Autodesk Inventor part; units mm, degrees
(part 2 of 5)
  spline S286 degree 2 poles (22.7063, 9.669) (22.5993, 9.5961) (22.4048, 9.5296) (22.2897, 9.5296) knots 0 0 0 1 2 2 2
  spline S287 degree 2 poles (22.2897, 9.5296) (22.1795, 9.5296) (21.9964, 9.5782) (21.904, 9.6479) knots 0 0 0 1 2 2 2
  spline S288 degree 2 poles (21.904, 9.6479) (21.797, 9.7306) (21.6868, 9.9818) (21.6868, 10.1585) knots 0 0 0 1 2 2 2
  spline S289 degree 2 poles (22.7128, 9.9883) (22.7128, 10.1909) (22.6382, 10.447) (22.5718, 10.5167) knots 0 0 0 1 2 2 2
  spline S290 degree 2 poles (22.5718, 10.5167) (22.5134, 10.5815) (22.3919, 10.6301) (22.3205, 10.6301) knots 0 0 0 1 2 2 2
  spline S291 degree 2 poles (22.3205, 10.6301) (22.1552, 10.6301) (21.9591, 10.3935) (21.9591, 10.1698) knots 0 0 0 1 2 2 2
  spline S292 degree 2 poles (21.9591, 10.1698) (21.9591, 10.0434) (22.0239, 9.8797) (22.0953, 9.8214) knots 0 0 0 1 2 2 2
  spline S293 degree 2 poles (22.0953, 9.8214) (22.1471, 9.7792) (22.2752, 9.7517) (22.3497, 9.7517) knots 0 0 0 1 2 2 2
  spline S294 degree 2 poles (22.3497, 9.7517) (22.4356, 9.7517) (22.6333, 9.8116) (22.7079, 9.8619) knots 0 0 0 1 2 2 2
  spline S295 degree 2 poles (22.7079, 9.8619) (22.7095, 9.8813) (22.7128, 9.9478) (22.7128, 9.9883) knots 0 0 0 1 2 2 2
  line L268 (24.0742, 10.8975) -> (23.2914, 8.374)
  line L269 (23.2914, 8.374) -> (23.0645, 8.374)
  line L270 (23.0645, 8.374) -> (23.844, 10.8975)
  line L271 (23.844, 10.8975) -> (24.0742, 10.8975)
  line L272 (25.528, 8.8084) -> (24.2946, 8.8084)
  line L273 (24.2946, 8.8084) -> (24.2946, 9.092)
  spline S296 degree 2 poles (24.2946, 9.092) (24.4275, 9.2168) (24.6641, 9.4486) (24.7776, 9.5734) knots 0 0 0 1 2 2 2
  spline S297 degree 2 poles (24.7776, 9.5734) (25.0061, 9.8246) (25.1731, 10.1261) (25.1731, 10.2865) knots 0 0 0 1 2 2 2
  spline S298 degree 2 poles (25.1731, 10.2865) (25.1731, 10.3708) (25.1212, 10.4972) (25.0742, 10.5377) knots 0 0 0 1 2 2 2
  spline S299 degree 2 poles (25.0742, 10.5377) (25.0272, 10.5782) (24.904, 10.6188) (24.8295, 10.6188) knots 0 0 0 1 2 2 2
  spline S300 degree 2 poles (24.8295, 10.6188) (24.7581, 10.6188) (24.6123, 10.5831) (24.5458, 10.5555) knots 0 0 0 1 2 2 2
  spline S301 degree 2 poles (24.5458, 10.5555) (24.4891, 10.5329) (24.3837, 10.468) (24.3513, 10.4453) knots 0 0 0 1 2 2 2
  line L274 (24.3513, 10.4453) -> (24.3367, 10.4453)
  line L275 (24.3367, 10.4453) -> (24.3367, 10.7306)
  spline S302 degree 2 poles (24.3367, 10.7306) (24.4194, 10.7711) (24.716, 10.8505) (24.8489, 10.8505) knots 0 0 0 1 2 2 2
  spline S303 degree 2 poles (24.8489, 10.8505) (25.1293, 10.8505) (25.4453, 10.5539) (25.4453, 10.3011) knots 0 0 0 1 2 2 2
  spline S304 degree 2 poles (25.4453, 10.3011) (25.4453, 10.1828) (25.3902, 9.985) (25.3416, 9.9008) knots 0 0 0 1 2 2 2
  spline S305 degree 2 poles (25.3416, 9.9008) (25.293, 9.8132) (25.152, 9.6414) (25.0742, 9.5588) knots 0 0 0 1 2 2 2
  spline S306 degree 2 poles (25.0742, 9.5588) (24.9478, 9.421) (24.6382, 9.1261) (24.5458, 9.0402) knots 0 0 0 1 2 2 2
  line L276 (24.5458, 9.0402) -> (25.528, 9.0402)
  line L277 (25.528, 9.0402) -> (25.528, 8.8084)
  spline S307 degree 2 poles (27.0401, 9.8084) (27.0401, 9.2703) (26.7273, 8.7662) (26.4016, 8.7662) knots 0 0 0 1 2 2 2
  spline S308 degree 2 poles (26.4016, 8.7662) (26.0709, 8.7662) (25.7614, 9.28) (25.7614, 9.8068) knots 0 0 0 1 2 2 2
  spline S309 degree 2 poles (25.7614, 9.8068) (25.7614, 10.3481) (26.0742, 10.8489) (26.4016, 10.8489) knots 0 0 0 1 2 2 2
  spline S310 degree 2 poles (26.4016, 10.8489) (26.7306, 10.8489) (27.0401, 10.3303) (27.0401, 9.8084) knots 0 0 0 1 2 2 2
  spline S311 degree 2 poles (26.6966, 9.199) (26.7354, 9.2978) (26.7679, 9.6026) (26.7679, 9.8084) knots 0 0 0 1 2 2 2
  spline S312 degree 2 poles (26.7679, 9.8084) (26.7679, 10.0142) (26.7354, 10.3173) (26.6949, 10.4194) knots 0 0 0 1 2 2 2
  spline S313 degree 2 poles (26.6949, 10.4194) (26.6544, 10.5215) (26.5134, 10.6269) (26.4016, 10.6269) knots 0 0 0 1 2 2 2
  spline S314 degree 2 poles (26.4016, 10.6269) (26.2897, 10.6269) (26.1455, 10.5215) (26.1034, 10.4162) knots 0 0 0 1 2 2 2
  spline S315 degree 2 poles (26.1034, 10.4162) (26.0628, 10.3141) (26.0337, 10.0029) (26.0337, 9.8068) knots 0 0 0 1 2 2 2
  spline S316 degree 2 poles (26.0337, 9.8068) (26.0337, 9.5961) (26.0596, 9.3141) (26.1017, 9.2038) knots 0 0 0 1 2 2 2
  spline S317 degree 2 poles (26.1017, 9.2038) (26.1406, 9.1001) (26.2849, 8.9883) (26.4016, 8.9883) knots 0 0 0 1 2 2 2
  spline S318 degree 2 poles (26.4016, 8.9883) (26.5118, 8.9883) (26.656, 9.0936) (26.6966, 9.199) knots 0 0 0 1 2 2 2
  spline S319 degree 2 poles (-27.8415, 6.1297) (-27.8415, 5.9806) (-27.955, 5.7521) (-28.049, 5.6775) knots 0 0 0 1 2 2 2
  spline S320 degree 2 poles (-28.049, 5.6775) (-28.1624, 5.59) (-28.4201, 5.5154) (-28.6244, 5.5154) knots 0 0 0 1 2 2 2
  line L278 (-28.6244, 5.5154) -> (-29.1981, 5.5154)
  line L279 (-29.1981, 5.5154) -> (-29.1981, 7.5154)
  line L280 (-29.1981, 7.5154) -> (-28.6681, 7.5154)
  spline S321 degree 2 poles (-28.6681, 7.5154) (-28.4542, 7.5154) (-28.2402, 7.4879) (-28.143, 7.4344) knots 0 0 0 1 2 2 2
  spline S322 degree 2 poles (-28.143, 7.4344) (-28.0344, 7.3777) (-27.9355, 7.1913) (-27.9355, 7.0649) knots 0 0 0 1 2 2 2
  spline S323 degree 2 poles (-27.9355, 7.0649) (-27.9355, 6.9239) (-28.0846, 6.7002) (-28.2159, 6.637) knots 0 0 0 1 2 2 2
  line L281 (-28.2159, 6.637) -> (-28.2159, 6.6273)
  spline S324 degree 2 poles (-28.2159, 6.6273) (-28.0376, 6.5786) (-27.8415, 6.3209) (-27.8415, 6.1297) knots 0 0 0 1 2 2 2
  spline S325 degree 2 poles (-28.1187, 6.1184) (-28.1187, 6.2318) (-28.1835, 6.3777) (-28.2808, 6.4295) knots 0 0 0 1 2 2 2
  spline S326 degree 2 poles (-28.2808, 6.4295) (-28.344, 6.462) (-28.4931, 6.4814) (-28.6308, 6.4814) knots 0 0 0 1 2 2 2
  line L282 (-28.6308, 6.4814) -> (-28.9323, 6.4814)
  line L283 (-28.9323, 6.4814) -> (-28.9323, 5.7423)
  line L284 (-28.9323, 5.7423) -> (-28.7167, 5.7423)
  spline S327 degree 2 poles (-28.7167, 5.7423) (-28.5417, 5.7423) (-28.3407, 5.7748) (-28.2629, 5.8266) knots 0 0 0 1 2 2 2
  spline S328 degree 2 poles (-28.2629, 5.8266) (-28.1884, 5.8801) (-28.1187, 6.013) (-28.1187, 6.1184) knots 0 0 0 1 2 2 2
  spline S329 degree 2 poles (-28.2127, 7.0276) (-28.2127, 7.0989) (-28.2613, 7.2059) (-28.3148, 7.2367) knots 0 0 0 1 2 2 2
  spline S330 degree 2 poles (-28.3148, 7.2367) (-28.3796, 7.2723) (-28.5368, 7.2885) (-28.6778, 7.2885) knots 0 0 0 1 2 2 2
  line L285 (-28.6778, 7.2885) -> (-28.9323, 7.2885)
  line L286 (-28.9323, 7.2885) -> (-28.9323, 6.7034)
  line L287 (-28.9323, 6.7034) -> (-28.6308, 6.7034)
  spline S331 degree 2 poles (-28.6308, 6.7034) (-28.506, 6.7034) (-28.3877, 6.7294) (-28.3245, 6.7699) knots 0 0 0 1 2 2 2
  spline S332 degree 2 poles (-28.3245, 6.7699) (-28.2629, 6.8088) (-28.2127, 6.9336) (-28.2127, 7.0276) knots 0 0 0 1 2 2 2
  spline S333 degree 2 poles (-26.7605, 5.6743) (-26.7913, 5.6516) (-26.895, 5.5705) (-26.9436, 5.5462) knots 0 0 0 1 2 2 2
  spline S334 degree 2 poles (-26.9436, 5.5462) (-27.0101, 5.5106) (-27.1349, 5.4733) (-27.2483, 5.4733) knots 0 0 0 1 2 2 2
  spline S335 degree 2 poles (-27.2483, 5.4733) (-27.3407, 5.4733) (-27.5077, 5.543) (-27.5709, 5.6062) knots 0 0 0 1 2 2 2
  spline S336 degree 2 poles (-27.5709, 5.6062) (-27.6308, 5.6678) (-27.7038, 5.8493) (-27.7038, 5.9498) knots 0 0 0 1 2 2 2
  spline S337 degree 2 poles (-27.7038, 5.9498) (-27.7038, 6.1054) (-27.5725, 6.3258) (-27.4299, 6.389) knots 0 0 0 1 2 2 2
  spline S338 degree 2 poles (-27.4299, 6.389) (-27.3034, 6.4474) (-26.9599, 6.4911) (-26.7605, 6.5025) knots 0 0 0 1 2 2 2
  line L288 (-26.7605, 6.5025) -> (-26.7605, 6.5511)
  spline S339 degree 2 poles (-26.7605, 6.5511) (-26.7605, 6.6386) (-26.814, 6.7472) (-26.8626, 6.778) knots 0 0 0 1 2 2 2
  spline S340 degree 2 poles (-26.8626, 6.778) (-26.9112, 6.8088) (-27.0506, 6.8282) (-27.1252, 6.8282) knots 0 0 0 1 2 2 2
  spline S341 degree 2 poles (-27.1252, 6.8282) (-27.2127, 6.8282) (-27.4493, 6.7764) (-27.5676, 6.7261) knots 0 0 0 1 2 2 2
  line L289 (-27.5676, 6.7261) -> (-27.5822, 6.7261)
  line L290 (-27.5822, 6.7261) -> (-27.5822, 6.9838)
  spline S342 degree 2 poles (-27.5822, 6.9838) (-27.5125, 7.0033) (-27.2516, 7.0519) (-27.1235, 7.0519) knots 0 0 0 1 2 2 2
  spline S343 degree 2 poles (-27.1235, 7.0519) (-26.968, 7.0519) (-26.7556, 7.0033) (-26.6714, 6.9401) knots 0 0 0 1 2 2 2
  spline S344 degree 2 poles (-26.6714, 6.9401) (-26.5887, 6.8785) (-26.5077, 6.6824) (-26.5077, 6.5414) knots 0 0 0 1 2 2 2
  line L291 (-26.5077, 6.5414) -> (-26.5077, 5.5154)
  line L292 (-26.5077, 5.5154) -> (-26.7605, 5.5154)
  line L293 (-26.7605, 5.5154) -> (-26.7605, 5.6743)
  line L294 (-26.7605, 5.885) -> (-26.7605, 6.3015)
  spline S345 degree 2 poles (-26.7605, 6.3015) (-26.8513, 6.2934) (-27.1252, 6.2658) (-27.2111, 6.2399) knots 0 0 0 1 2 2 2
  spline S346 degree 2 poles (-27.2111, 6.2399) (-27.3116, 6.2091) (-27.4428, 6.0811) (-27.4428, 5.9676) knots 0 0 0 1 2 2 2
  spline S347 degree 2 poles (-27.4428, 5.9676) (-27.4428, 5.838) (-27.297, 5.7067) (-27.1576, 5.7067) knots 0 0 0 1 2 2 2
  spline S348 degree 2 poles (-27.1576, 5.7067) (-27.0393, 5.7067) (-26.8448, 5.8088) (-26.7605, 5.885) knots 0 0 0 1 2 2 2
  line L295 (-24.9744, 5.5154) -> (-25.2273, 5.5154)
  line L296 (-25.2273, 5.5154) -> (-25.2273, 6.3712)
  spline S349 degree 2 poles (-25.2273, 6.3712) (-25.2273, 6.4749) (-25.2467, 6.6532) (-25.2759, 6.7067) knots 0 0 0 1 2 2 2
  spline S350 degree 2 poles (-25.2759, 6.7067) (-25.3067, 6.7634) (-25.4169, 6.8185) (-25.5109, 6.8185) knots 0 0 0 1 2 2 2
  spline S351 degree 2 poles (-25.5109, 6.8185) (-25.6049, 6.8185) (-25.8043, 6.718) (-25.8999, 6.637) knots 0 0 0 1 2 2 2
  line L297 (-25.8999, 6.637) -> (-25.8999, 5.5154)
  line L298 (-25.8999, 5.5154) -> (-26.1527, 5.5154)
  line L299 (-26.1527, 5.5154) -> (-26.1527, 7.0162)
  line L300 (-26.1527, 7.0162) -> (-25.8999, 7.0162)
  line L301 (-25.8999, 7.0162) -> (-25.8999, 6.8493)
  spline S352 degree 2 poles (-25.8999, 6.8493) (-25.7864, 6.9514) (-25.5676, 7.0584) (-25.4445, 7.0584) knots 0 0 0 1 2 2 2
  spline S353 degree 2 poles (-25.4445, 7.0584) (-25.224, 7.0584) (-24.9744, 6.7667) (-24.9744, 6.4895) knots 0 0 0 1 2 2 2
  line L302 (-24.9744, 6.4895) -> (-24.9744, 5.5154)
  spline S354 degree 2 poles (-24.0231, 5.4814) (-24.1787, 5.4814) (-24.4364, 5.577) (-24.5287, 5.6743) knots 0 0 0 1 2 2 2
  spline S355 degree 2 poles (-24.5287, 5.6743) (-24.6211, 5.7699) (-24.7232, 6.0649) (-24.7232, 6.2626) knots 0 0 0 1 2 2 2
  spline S356 degree 2 poles (-24.7232, 6.2626) (-24.7232, 6.4603) (-24.6179, 6.7488) (-24.5287, 6.8461) knots 0 0 0 1 2 2 2
  spline S357 degree 2 poles (-24.5287, 6.8461) (-24.4396, 6.9449) (-24.1754, 7.0503) (-24.0231, 7.0503) knots 0 0 0 1 2 2 2
  spline S358 degree 2 poles (-24.0231, 7.0503) (-23.8999, 7.0503) (-23.6697, 6.9806) (-23.5806, 6.9352) knots 0 0 0 1 2 2 2
  line L303 (-23.5806, 6.9352) -> (-23.5806, 6.6516)
  line L304 (-23.5806, 6.6516) -> (-23.5952, 6.6516)
  spline S359 degree 2 poles (-23.5952, 6.6516) (-23.6227, 6.6743) (-23.707, 6.7326) (-23.767, 6.7634) knots 0 0 0 1 2 2 2
  spline S360 degree 2 poles (-23.767, 6.7634) (-23.8205, 6.7893) (-23.9631, 6.8299) (-24.0279, 6.8299) knots 0 0 0 1 2 2 2
  spline S361 degree 2 poles (-24.0279, 6.8299) (-24.224, 6.8299) (-24.4623, 6.5333) (-24.4623, 6.2626) knots 0 0 0 1 2 2 2
  spline S362 degree 2 poles (-24.4623, 6.2626) (-24.4623, 5.9984) (-24.2321, 5.7018) (-24.0279, 5.7018) knots 0 0 0 1 2 2 2
  spline S363 degree 2 poles (-24.0279, 5.7018) (-23.9047, 5.7018) (-23.6811, 5.8039) (-23.5952, 5.8833) knots 0 0 0 1 2 2 2
  line L305 (-23.5952, 5.8833) -> (-23.5806, 5.8833)
  line L306 (-23.5806, 5.8833) -> (-23.5806, 5.5997)
  spline S364 degree 2 poles (-23.5806, 5.5997) (-23.6179, 5.5819) (-23.7313, 5.5316) (-23.7767, 5.5203) knots 0 0 0 1 2 2 2
  spline S365 degree 2 poles (-23.7767, 5.5203) (-23.8415, 5.5009) (-23.9436, 5.4814) (-24.0231, 5.4814) knots 0 0 0 1 2 2 2
  spline S366 degree 2 poles (-22.1171, 6.2658) (-22.1171, 5.8866) (-22.4817, 5.4733) (-22.7864, 5.4733) knots 0 0 0 1 2 2 2
  spline S367 degree 2 poles (-22.7864, 5.4733) (-23.0992, 5.4733) (-23.4574, 5.8996) (-23.4574, 6.2658) knots 0 0 0 1 2 2 2
  spline S368 degree 2 poles (-23.4574, 6.2658) (-23.4574, 6.6419) (-23.0879, 7.0584) (-22.7864, 7.0584) knots 0 0 0 1 2 2 2
  spline S369 degree 2 poles (-22.7864, 7.0584) (-22.4817, 7.0584) (-22.1171, 6.6435) (-22.1171, 6.2658) knots 0 0 0 1 2 2 2
  spline S370 degree 2 poles (-22.378, 6.2658) (-22.378, 6.5576) (-22.5903, 6.8412) (-22.7864, 6.8412) knots 0 0 0 1 2 2 2
  spline S371 degree 2 poles (-22.7864, 6.8412) (-22.9825, 6.8412) (-23.1965, 6.5576) (-23.1965, 6.2658) knots 0 0 0 1 2 2 2
  spline S372 degree 2 poles (-23.1965, 6.2658) (-23.1965, 5.9822) (-22.9825, 5.6905) (-22.7864, 5.6905) knots 0 0 0 1 2 2 2
  spline S373 degree 2 poles (-22.7864, 5.6905) (-22.5919, 5.6905) (-22.378, 5.9774) (-22.378, 6.2658) knots 0 0 0 1 2 2 2
  line L307 (-19.8448, 5.5154) -> (-20.0976, 5.5154)
  line L308 (-20.0976, 5.5154) -> (-20.0976, 5.6678)
  spline S374 degree 2 poles (-20.0976, 5.6678) (-20.156, 5.6192) (-20.2419, 5.5543) (-20.3002, 5.5268) knots 0 0 0 1 2 2 2
  spline S375 degree 2 poles (-20.3002, 5.5268) (-20.3537, 5.5009) (-20.4688, 5.4733) (-20.5449, 5.4733) knots 0 0 0 1 2 2 2
  spline S376 degree 2 poles (-20.5449, 5.4733) (-20.6681, 5.4733) (-20.8756, 5.5754) (-20.9485, 5.6743) knots 0 0 0 1 2 2 2
  spline S377 degree 2 poles (-20.9485, 5.6743) (-21.0214, 5.7731) (-21.1025, 6.0649) (-21.1025, 6.2545) knots 0 0 0 1 2 2 2
  spline S378 degree 2 poles (-21.1025, 6.2545) (-21.1025, 6.4522) (-21.0004, 6.7407) (-20.9112, 6.8493) knots 0 0 0 1 2 2 2
  spline S379 degree 2 poles (-20.9112, 6.8493) (-20.8286, 6.9466) (-20.5968, 7.0584) (-20.4688, 7.0584) knots 0 0 0 1 2 2 2
  spline S380 degree 2 poles (-20.4688, 7.0584) (-20.3569, 7.0584) (-20.19, 7.0081) (-20.0976, 6.9563) knots 0 0 0 1 2 2 2
  line L309 (-20.0976, 6.9563) -> (-20.0976, 7.6046)
  line L310 (-20.0976, 7.6046) -> (-19.8448, 7.6046)
  line L311 (-19.8448, 7.6046) -> (-19.8448, 5.5154)
  line L312 (-20.0976, 5.8801) -> (-20.0976, 6.7472)
  spline S381 degree 2 poles (-20.0976, 6.7472) (-20.1916, 6.7926) (-20.3407, 6.8266) (-20.4266, 6.8266) knots 0 0 0 1 2 2 2
  spline S382 degree 2 poles (-20.4266, 6.8266) (-20.6211, 6.8266) (-20.8415, 6.5349) (-20.8415, 6.2594) knots 0 0 0 1 2 2 2
  spline S383 degree 2 poles (-20.8415, 6.2594) (-20.8415, 5.9936) (-20.673, 5.7132) (-20.4866, 5.7132) knots 0 0 0 1 2 2 2
  spline S384 degree 2 poles (-20.4866, 5.7132) (-20.3877, 5.7132) (-20.1868, 5.8039) (-20.0976, 5.8801) knots 0 0 0 1 2 2 2
  line L313 (-19.2208, 5.5154) -> (-19.4736, 5.5154)
  line L314 (-19.4736, 5.5154) -> (-19.4736, 7.0162)
  line L315 (-19.4736, 7.0162) -> (-19.2208, 7.0162)
  line L316 (-19.2208, 7.0162) -> (-19.2208, 5.5154)
  line L317 (-19.203, 7.2658) -> (-19.4898, 7.2658)
  line L318 (-19.4898, 7.2658) -> (-19.4898, 7.5284)
  line L319 (-19.4898, 7.5284) -> (-19.203, 7.5284)
  line L320 (-19.203, 7.5284) -> (-19.203, 7.2658)
  spline S385 degree 2 poles (-16.7329, 6.3064) (-16.7329, 5.9303) (-17.0911, 5.4863) (-17.365, 5.4863) knots 0 0 0 1 2 2 2
  spline S386 degree 2 poles (-17.365, 5.4863) (-17.4769, 5.4863) (-17.6487, 5.5381) (-17.7378, 5.5916) knots 0 0 0 1 2 2 2
  line L321 (-17.7378, 5.5916) -> (-17.7378, 4.9628)
  line L322 (-17.7378, 4.9628) -> (-17.9906, 4.9628)
  line L323 (-17.9906, 4.9628) -> (-17.9906, 7.0162)
  line L324 (-17.9906, 7.0162) -> (-17.7378, 7.0162)
  line L325 (-17.7378, 7.0162) -> (-17.7378, 6.859)
  spline S387 degree 2 poles (-17.7378, 6.859) (-17.6438, 6.9449) (-17.4137, 7.0584) (-17.2791, 7.0584) knots 0 0 0 1 2 2 2
  spline S388 degree 2 poles (-17.2791, 7.0584) (-17.0214, 7.0584) (-16.7329, 6.65) (-16.7329, 6.3064) knots 0 0 0 1 2 2 2
  spline S389 degree 2 poles (-16.9939, 6.2772) (-16.9939, 6.5349) (-17.1576, 6.8185) (-17.3407, 6.8185) knots 0 0 0 1 2 2 2
  spline S390 degree 2 poles (-17.3407, 6.8185) (-17.4477, 6.8185) (-17.6487, 6.7229) (-17.7378, 6.6483) knots 0 0 0 1 2 2 2
  line L326 (-17.7378, 6.6483) -> (-17.7378, 5.7958)
  spline S391 degree 2 poles (-17.7378, 5.7958) (-17.6389, 5.7488) (-17.4979, 5.7132) (-17.4072, 5.7132) knots 0 0 0 1 2 2 2
  spline S392 degree 2 poles (-17.4072, 5.7132) (-17.2111, 5.7132) (-16.9939, 6.0017) (-16.9939, 6.2772) knots 0 0 0 1 2 2 2
  line L327 (-15.6746, 6.7456) -> (-15.6876, 6.7456)
  spline S393 degree 2 poles (-15.6876, 6.7456) (-15.7167, 6.7537) (-15.7799, 6.7569) (-15.8237, 6.7569) knots 0 0 0 1 2 2 2
  spline S394 degree 2 poles (-15.8237, 6.7569) (-15.9258, 6.7569) (-16.1268, 6.6678) (-16.2175, 6.5803) knots 0 0 0 1 2 2 2
  line L328 (-16.2175, 6.5803) -> (-16.2175, 5.5154)
  line L329 (-16.2175, 5.5154) -> (-16.4704, 5.5154)
  line L330 (-16.4704, 5.5154) -> (-16.4704, 7.0162)
  line L331 (-16.4704, 7.0162) -> (-16.2175, 7.0162)
  line L332 (-16.2175, 7.0162) -> (-16.2175, 6.7926)
  spline S395 degree 2 poles (-16.2175, 6.7926) (-16.0798, 6.9158) (-15.874, 7.0162) (-15.7767, 7.0162) knots 0 0 0 1 2 2 2
  spline S396 degree 2 poles (-15.7767, 7.0162) (-15.7378, 7.0162) (-15.6989, 7.013) (-15.6746, 7.0081) knots 0 0 0 1 2 2 2
  line L333 (-15.6746, 7.0081) -> (-15.6746, 6.7456)
  spline S397 degree 2 poles (-14.2451, 6.2658) (-14.2451, 5.8866) (-14.6098, 5.4733) (-14.9145, 5.4733) knots 0 0 0 1 2 2 2
  spline S398 degree 2 poles (-14.9145, 5.4733) (-15.2273, 5.4733) (-15.5855, 5.8996) (-15.5855, 6.2658) knots 0 0 0 1 2 2 2
  spline S399 degree 2 poles (-15.5855, 6.2658) (-15.5855, 6.6419) (-15.2159, 7.0584) (-14.9145, 7.0584) knots 0 0 0 1 2 2 2
  spline S400 degree 2 poles (-14.9145, 7.0584) (-14.6098, 7.0584) (-14.2451, 6.6435) (-14.2451, 6.2658) knots 0 0 0 1 2 2 2
  spline S401 degree 2 poles (-14.506, 6.2658) (-14.506, 6.5576) (-14.7184, 6.8412) (-14.9145, 6.8412) knots 0 0 0 1 2 2 2
  spline S402 degree 2 poles (-14.9145, 6.8412) (-15.1106, 6.8412) (-15.3245, 6.5576) (-15.3245, 6.2658) knots 0 0 0 1 2 2 2
  spline S403 degree 2 poles (-15.3245, 6.2658) (-15.3245, 5.9822) (-15.1106, 5.6905) (-14.9145, 5.6905) knots 0 0 0 1 2 2 2
  spline S404 degree 2 poles (-14.9145, 5.6905) (-14.72, 5.6905) (-14.506, 5.9774) (-14.506, 6.2658) knots 0 0 0 1 2 2 2
  line L334 (-12.8075, 7.0162) -> (-13.3731, 5.5154)
  line L335 (-13.3731, 5.5154) -> (-13.6, 5.5154)
  line L336 (-13.6, 5.5154) -> (-14.1608, 7.0162)
  line L337 (-14.1608, 7.0162) -> (-13.8869, 7.0162)
  line L338 (-13.8869, 7.0162) -> (-13.4769, 5.8607)
  line L339 (-13.4769, 5.8607) -> (-13.0701, 7.0162)
  line L340 (-13.0701, 7.0162) -> (-12.8075, 7.0162)
  spline S405 degree 2 poles (-11.7799, 5.6743) (-11.8107, 5.6516) (-11.9145, 5.5705) (-11.9631, 5.5462) knots 0 0 0 1 2 2 2
  spline S406 degree 2 poles (-11.9631, 5.5462) (-12.0295, 5.5106) (-12.1543, 5.4733) (-12.2678, 5.4733) knots 0 0 0 1 2 2 2
  spline S407 degree 2 poles (-12.2678, 5.4733) (-12.3602, 5.4733) (-12.5271, 5.543) (-12.5903, 5.6062) knots 0 0 0 1 2 2 2
  spline S408 degree 2 poles (-12.5903, 5.6062) (-12.6503, 5.6678) (-12.7232, 5.8493) (-12.7232, 5.9498) knots 0 0 0 1 2 2 2
  spline S409 degree 2 poles (-12.7232, 5.9498) (-12.7232, 6.1054) (-12.5919, 6.3258) (-12.4493, 6.389) knots 0 0 0 1 2 2 2
  spline S410 degree 2 poles (-12.4493, 6.389) (-12.3229, 6.4474) (-11.9793, 6.4911) (-11.7799, 6.5025) knots 0 0 0 1 2 2 2
  line L341 (-11.7799, 6.5025) -> (-11.7799, 6.5511)
  spline S411 degree 2 poles (-11.7799, 6.5511) (-11.7799, 6.6386) (-11.8334, 6.7472) (-11.8821, 6.778) knots 0 0 0 1 2 2 2
  spline S412 degree 2 poles (-11.8821, 6.778) (-11.9307, 6.8088) (-12.0701, 6.8282) (-12.1446, 6.8282) knots 0 0 0 1 2 2 2
  spline S413 degree 2 poles (-12.1446, 6.8282) (-12.2321, 6.8282) (-12.4688, 6.7764) (-12.5871, 6.7261) knots 0 0 0 1 2 2 2
  line L342 (-12.5871, 6.7261) -> (-12.6017, 6.7261)
  line L343 (-12.6017, 6.7261) -> (-12.6017, 6.9838)
  spline S414 degree 2 poles (-12.6017, 6.9838) (-12.532, 7.0033) (-12.271, 7.0519) (-12.143, 7.0519) knots 0 0 0 1 2 2 2
  spline S415 degree 2 poles (-12.143, 7.0519) (-11.9874, 7.0519) (-11.7751, 7.0033) (-11.6908, 6.9401) knots 0 0 0 1 2 2 2
  spline S416 degree 2 poles (-11.6908, 6.9401) (-11.6081, 6.8785) (-11.5271, 6.6824) (-11.5271, 6.5414) knots 0 0 0 1 2 2 2
  line L344 (-11.5271, 6.5414) -> (-11.5271, 5.5154)
  line L345 (-11.5271, 5.5154) -> (-11.7799, 5.5154)
  line L346 (-11.7799, 5.5154) -> (-11.7799, 5.6743)
  line L347 (-11.7799, 5.885) -> (-11.7799, 6.3015)
  spline S417 degree 2 poles (-11.7799, 6.3015) (-11.8707, 6.2934) (-12.1446, 6.2658) (-12.2305, 6.2399) knots 0 0 0 1 2 2 2
  spline S418 degree 2 poles (-12.2305, 6.2399) (-12.331, 6.2091) (-12.4623, 6.0811) (-12.4623, 5.9676) knots 0 0 0 1 2 2 2
  spline S419 degree 2 poles (-12.4623, 5.9676) (-12.4623, 5.838) (-12.3164, 5.7067) (-12.177, 5.7067) knots 0 0 0 1 2 2 2
  spline S420 degree 2 poles (-12.177, 5.7067) (-12.0587, 5.7067) (-11.8642, 5.8088) (-11.7799, 5.885) knots 0 0 0 1 2 2 2
  spline S421 degree 2 poles (-9.0555, 6.3064) (-9.0555, 5.9303) (-9.4137, 5.4863) (-9.6876, 5.4863) knots 0 0 0 1 2 2 2
  spline S422 degree 2 poles (-9.6876, 5.4863) (-9.7994, 5.4863) (-9.9712, 5.5381) (-10.0603, 5.5916) knots 0 0 0 1 2 2 2
  line L348 (-10.0603, 5.5916) -> (-10.0603, 4.9628)
  line L349 (-10.0603, 4.9628) -> (-10.3132, 4.9628)
  line L350 (-10.3132, 4.9628) -> (-10.3132, 7.0162)
  line L351 (-10.3132, 7.0162) -> (-10.0603, 7.0162)
  line L352 (-10.0603, 7.0162) -> (-10.0603, 6.859)
  spline S423 degree 2 poles (-10.0603, 6.859) (-9.9663, 6.9449) (-9.7362, 7.0584) (-9.6017, 7.0584) knots 0 0 0 1 2 2 2
  spline S424 degree 2 poles (-9.6017, 7.0584) (-9.344, 7.0584) (-9.0555, 6.65) (-9.0555, 6.3064) knots 0 0 0 1 2 2 2
  spline S425 degree 2 poles (-9.3164, 6.2772) (-9.3164, 6.5349) (-9.4801, 6.8185) (-9.6633, 6.8185) knots 0 0 0 1 2 2 2
  spline S426 degree 2 poles (-9.6633, 6.8185) (-9.7702, 6.8185) (-9.9712, 6.7229) (-10.0603, 6.6483) knots 0 0 0 1 2 2 2
  line L353 (-10.0603, 6.6483) -> (-10.0603, 5.7958)
  spline S427 degree 2 poles (-10.0603, 5.7958) (-9.9615, 5.7488) (-9.8205, 5.7132) (-9.7297, 5.7132) knots 0 0 0 1 2 2 2
  spline S428 degree 2 poles (-9.7297, 5.7132) (-9.5336, 5.7132) (-9.3164, 6.0017) (-9.3164, 6.2772) knots 0 0 0 1 2 2 2
  spline S429 degree 2 poles (-8.1414, 5.4814) (-8.5012, 5.4814) (-8.8966, 5.885) (-8.8966, 6.2577) knots 0 0 0 1 2 2 2
  spline S430 degree 2 poles (-8.8966, 6.2577) (-8.8966, 6.624) (-8.5125, 7.0584) (-8.203, 7.0584) knots 0 0 0 1 2 2 2
  spline S431 degree 2 poles (-8.203, 7.0584) (-8.0636, 7.0584) (-7.848, 6.9774) (-7.7686, 6.8915) knots 0 0 0 1 2 2 2
  spline S432 degree 2 poles (-7.7686, 6.8915) (-7.6876, 6.8056) (-7.6017, 6.5576) (-7.6017, 6.3777) knots 0 0 0 1 2 2 2
  line L354 (-7.6017, 6.3777) -> (-7.6017, 6.2399)
  line L355 (-7.6017, 6.2399) -> (-8.6406, 6.2399)
  spline S433 degree 2 poles (-8.6406, 6.2399) (-8.6406, 5.979) (-8.378, 5.7018) (-8.1446, 5.7018) knots 0 0 0 1 2 2 2
  spline S434 degree 2 poles (-8.1446, 5.7018) (-8.062, 5.7018) (-7.9015, 5.7391) (-7.8367, 5.7683) knots 0 0 0 1 2 2 2
  spline S435 degree 2 poles (-7.8367, 5.7683) (-7.7686, 5.8007) (-7.6746, 5.8574) (-7.6438, 5.8833) knots 0 0 0 1 2 2 2
  line L356 (-7.6438, 5.8833) -> (-7.6292, 5.8833)
  line L357 (-7.6292, 5.8833) -> (-7.6292, 5.6078)
  spline S436 degree 2 poles (-7.6292, 5.6078) (-7.673, 5.59) (-7.8059, 5.5381) (-7.8577, 5.5235) knots 0 0 0 1 2 2 2
  spline S437 degree 2 poles (-7.8577, 5.5235) (-7.9307, 5.5025) (-8.0506, 5.4814) (-8.1414, 5.4814) knots 0 0 0 1 2 2 2
  spline S438 degree 2 poles (-7.848, 6.4328) (-7.8513, 6.5349) (-7.8934, 6.684) (-7.9339, 6.7342) knots 0 0 0 1 2 2 2
  spline S439 degree 2 poles (-7.9339, 6.7342) (-7.9777, 6.791) (-8.1154, 6.8509) (-8.2175, 6.8509) knots 0 0 0 1 2 2 2
  spline S440 degree 2 poles (-8.2175, 6.8509) (-8.318, 6.8509) (-8.459, 6.791) (-8.5174, 6.7326) knots 0 0 0 1 2 2 2
  spline S441 degree 2 poles (-8.5174, 6.7326) (-8.5741, 6.6727) (-8.6325, 6.5284) (-8.6406, 6.4328) knots 0 0 0 1 2 2 2
  line L358 (-8.6406, 6.4328) -> (-7.848, 6.4328)
  line L359 (-6.5498, 6.7456) -> (-6.5628, 6.7456)
  spline S442 degree 2 poles (-6.5628, 6.7456) (-6.5919, 6.7537) (-6.6552, 6.7569) (-6.6989, 6.7569) knots 0 0 0 1 2 2 2
  spline S443 degree 2 poles (-6.6989, 6.7569) (-6.801, 6.7569) (-7.002, 6.6678) (-7.0928, 6.5803) knots 0 0 0 1 2 2 2
  line L360 (-7.0928, 6.5803) -> (-7.0928, 5.5154)
  line L361 (-7.0928, 5.5154) -> (-7.3456, 5.5154)
  line L362 (-7.3456, 5.5154) -> (-7.3456, 7.0162)
  line L363 (-7.3456, 7.0162) -> (-7.0928, 7.0162)
  line L364 (-7.0928, 7.0162) -> (-7.0928, 6.7926)
  spline S444 degree 2 poles (-7.0928, 6.7926) (-6.955, 6.9158) (-6.7492, 7.0162) (-6.6519, 7.0162) knots 0 0 0 1 2 2 2
  spline S445 degree 2 poles (-6.6519, 7.0162) (-6.613, 7.0162) (-6.5741, 7.013) (-6.5498, 7.0081) knots 0 0 0 1 2 2 2
  line L365 (-6.5498, 7.0081) -> (-6.5498, 6.7456)
  line L366 (-3.7929, 5.5154) -> (-3.7929, 6.3842)
  spline S446 degree 2 poles (-3.7929, 6.3842) (-3.7929, 6.4879) (-3.8091, 6.6645) (-3.8351, 6.7132) knots 0 0 0 1 2 2 2
  spline S447 degree 2 poles (-3.8351, 6.7132) (-3.861, 6.7667) (-3.9599, 6.8185) (-4.0458, 6.8185) knots 0 0 0 1 2 2 2
  spline S448 degree 2 poles (-4.0458, 6.8185) (-4.1235, 6.8185) (-4.3018, 6.7229) (-4.3958, 6.6321) knots 0 0 0 1 2 2 2
  spline S449 degree 2 poles (-4.3958, 6.6321) (-4.3942, 6.6094) (-4.391, 6.5462) (-4.391, 6.5041) knots 0 0 0 1 2 2 2
  line L367 (-4.391, 6.5041) -> (-4.391, 5.5154)
  line L368 (-4.391, 5.5154) -> (-4.6438, 5.5154)
  line L369 (-4.6438, 5.5154) -> (-4.6438, 6.3842)
  spline S450 degree 2 poles (-4.6438, 6.3842) (-4.6438, 6.4879) (-4.66, 6.6645) (-4.6859, 6.7132) knots 0 0 0 1 2 2 2
  spline S451 degree 2 poles (-4.6859, 6.7132) (-4.7119, 6.7667) (-4.8107, 6.8185) (-4.8966, 6.8185) knots 0 0 0 1 2 2 2
  spline S452 degree 2 poles (-4.8966, 6.8185) (-4.9777, 6.8185) (-5.1576, 6.7164) (-5.2419, 6.637) knots 0 0 0 1 2 2 2
  line L370 (-5.2419, 6.637) -> (-5.2419, 5.5154)
  line L371 (-5.2419, 5.5154) -> (-5.4947, 5.5154)
  line L372 (-5.4947, 5.5154) -> (-5.4947, 7.0162)
  line L373 (-5.4947, 7.0162) -> (-5.2419, 7.0162)
  line L374 (-5.2419, 7.0162) -> (-5.2419, 6.8509)
  spline S453 degree 2 poles (-5.2419, 6.8509) (-5.143, 6.9498) (-4.9485, 7.0584) (-4.8318, 7.0584) knots 0 0 0 1 2 2 2
  spline S454 degree 2 poles (-4.8318, 7.0584) (-4.6989, 7.0584) (-4.4931, 6.9368) (-4.4396, 6.7991) knots 0 0 0 1 2 2 2
  spline S455 degree 2 poles (-4.4396, 6.7991) (-4.3245, 6.9271) (-4.1073, 7.0584) (-3.9809, 7.0584) knots 0 0 0 1 2 2 2
  spline S456 degree 2 poles (-3.9809, 7.0584) (-3.8837, 7.0584) (-3.7248, 6.9984) (-3.6665, 6.9303) knots 0 0 0 1 2 2 2
  spline S457 degree 2 poles (-3.6665, 6.9303) (-3.6065, 6.8623) (-3.5401, 6.6581) (-3.5401, 6.5041) knots 0 0 0 1 2 2 2
  line L375 (-3.5401, 6.5041) -> (-3.5401, 5.5154)
  line L376 (-3.5401, 5.5154) -> (-3.7929, 5.5154)
  spline S458 degree 2 poles (-1.9517, 6.2658) (-1.9517, 5.8866) (-2.3164, 5.4733) (-2.6211, 5.4733) knots 0 0 0 1 2 2 2
  spline S459 degree 2 poles (-2.6211, 5.4733) (-2.9339, 5.4733) (-3.2921, 5.8996) (-3.2921, 6.2658) knots 0 0 0 1 2 2 2
  spline S460 degree 2 poles (-3.2921, 6.2658) (-3.2921, 6.6419) (-2.9226, 7.0584) (-2.6211, 7.0584) knots 0 0 0 1 2 2 2
  spline S461 degree 2 poles (-2.6211, 7.0584) (-2.3164, 7.0584) (-1.9517, 6.6435) (-1.9517, 6.2658) knots 0 0 0 1 2 2 2
  spline S462 degree 2 poles (-2.2127, 6.2658) (-2.2127, 6.5576) (-2.425, 6.8412) (-2.6211, 6.8412) knots 0 0 0 1 2 2 2
  spline S463 degree 2 poles (-2.6211, 6.8412) (-2.8172, 6.8412) (-3.0312, 6.5576) (-3.0312, 6.2658) knots 0 0 0 1 2 2 2
  spline S464 degree 2 poles (-3.0312, 6.2658) (-3.0312, 5.9822) (-2.8172, 5.6905) (-2.6211, 5.6905) knots 0 0 0 1 2 2 2
  spline S465 degree 2 poles (-2.6211, 5.6905) (-2.4266, 5.6905) (-2.2127, 5.9774) (-2.2127, 6.2658) knots 0 0 0 1 2 2 2
  spline S466 degree 2 poles (-1.2386, 5.4863) (-1.4445, 5.4863) (-1.6762, 5.7213) (-1.6762, 5.9757) knots 0 0 0 1 2 2 2
  line L377 (-1.6762, 5.9757) -> (-1.6762, 6.8072)
  line L378 (-1.6762, 6.8072) -> (-1.8464, 6.8072)
  line L379 (-1.8464, 6.8072) -> (-1.8464, 7.0162)
  line L380 (-1.8464, 7.0162) -> (-1.6762, 7.0162)
  line L381 (-1.6762, 7.0162) -> (-1.6762, 7.4474)
  line L382 (-1.6762, 7.4474) -> (-1.4234, 7.4474)
  line L383 (-1.4234, 7.4474) -> (-1.4234, 7.0162)
  line L384 (-1.4234, 7.0162) -> (-0.9582, 7.0162)
  line L385 (-0.9582, 7.0162) -> (-0.9582, 6.8072)
  line L386 (-0.9582, 6.8072) -> (-1.4234, 6.8072)
  line L387 (-1.4234, 6.8072) -> (-1.4234, 6.0924)
  spline S467 degree 2 poles (-1.4234, 6.0924) (-1.4234, 5.979) (-1.4153, 5.8542) (-1.3877, 5.8007) knots 0 0 0 1 2 2 2
  spline S468 degree 2 poles (-1.3877, 5.8007) (-1.365, 5.7537) (-1.2629, 5.7067) (-1.1754, 5.7067) knots 0 0 0 1 2 2 2
  spline S469 degree 2 poles (-1.1754, 5.7067) (-1.1138, 5.7067) (-0.9987, 5.744) (-0.9728, 5.7553) knots 0 0 0 1 2 2 2
  line L388 (-0.9728, 5.7553) -> (-0.9582, 5.7553)
  line L389 (-0.9582, 5.7553) -> (-0.9582, 5.5284)
  spline S470 degree 2 poles (-0.9582, 5.5284) (-1.0295, 5.509) (-1.1754, 5.4863) (-1.2386, 5.4863) knots 0 0 0 1 2 2 2
  spline S471 degree 2 poles (0.4615, 6.2658) (0.4615, 5.8866) (0.0969, 5.4733) (-0.2078, 5.4733) knots 0 0 0 1 2 2 2
  spline S472 degree 2 poles (-0.2078, 5.4733) (-0.5206, 5.4733) (-0.8788, 5.8996) (-0.8788, 6.2658) knots 0 0 0 1 2 2 2
  spline S473 degree 2 poles (-0.8788, 6.2658) (-0.8788, 6.6419) (-0.5093, 7.0584) (-0.2078, 7.0584) knots 0 0 0 1 2 2 2
  spline S474 degree 2 poles (-0.2078, 7.0584) (0.0969, 7.0584) (0.4615, 6.6435) (0.4615, 6.2658) knots 0 0 0 1 2 2 2
  spline S475 degree 2 poles (0.2006, 6.2658) (0.2006, 6.5576) (-0.0117, 6.8412) (-0.2078, 6.8412) knots 0 0 0 1 2 2 2
  spline S476 degree 2 poles (-0.2078, 6.8412) (-0.4039, 6.8412) (-0.6179, 6.5576) (-0.6179, 6.2658) knots 0 0 0 1 2 2 2
  spline S477 degree 2 poles (-0.6179, 6.2658) (-0.6179, 5.9822) (-0.4039, 5.6905) (-0.2078, 5.6905) knots 0 0 0 1 2 2 2
  spline S478 degree 2 poles (-0.2078, 5.6905) (-0.0133, 5.6905) (0.2006, 5.9774) (0.2006, 6.2658) knots 0 0 0 1 2 2 2
  line L390 (1.5166, 6.7456) -> (1.5037, 6.7456)
  spline S479 degree 2 poles (1.5037, 6.7456) (1.4745, 6.7537) (1.4113, 6.7569) (1.3675, 6.7569) knots 0 0 0 1 2 2 2
  spline S480 degree 2 poles (1.3675, 6.7569) (1.2654, 6.7569) (1.0645, 6.6678) (0.9737, 6.5803) knots 0 0 0 1 2 2 2
  line L391 (0.9737, 6.5803) -> (0.9737, 5.5154)
  line L392 (0.9737, 5.5154) -> (0.7209, 5.5154)
  line L393 (0.7209, 5.5154) -> (0.7209, 7.0162)
  line L394 (0.7209, 7.0162) -> (0.9737, 7.0162)
  line L395 (0.9737, 7.0162) -> (0.9737, 6.7926)
  spline S481 degree 2 poles (0.9737, 6.7926) (1.1115, 6.9158) (1.3173, 7.0162) (1.4145, 7.0162) knots 0 0 0 1 2 2 2
  spline S482 degree 2 poles (1.4145, 7.0162) (1.4534, 7.0162) (1.4923, 7.013) (1.5166, 7.0081) knots 0 0 0 1 2 2 2
  line L396 (1.5166, 7.0081) -> (1.5166, 6.7456)
  spline S483 degree 2 poles (2.3643, 5.4814) (2.0045, 5.4814) (1.609, 5.885) (1.609, 6.2577) knots 0 0 0 1 2 2 2
  spline S484 degree 2 poles (1.609, 6.2577) (1.609, 6.624) (1.9931, 7.0584) (2.3027, 7.0584) knots 0 0 0 1 2 2 2
  spline S485 degree 2 poles (2.3027, 7.0584) (2.4421, 7.0584) (2.6577, 6.9774) (2.7371, 6.8915) knots 0 0 0 1 2 2 2
  spline S486 degree 2 poles (2.7371, 6.8915) (2.8181, 6.8056) (2.904, 6.5576) (2.904, 6.3777) knots 0 0 0 1 2 2 2
  line L397 (2.904, 6.3777) -> (2.904, 6.2399)
  line L398 (2.904, 6.2399) -> (1.8651, 6.2399)
  spline S487 degree 2 poles (1.8651, 6.2399) (1.8651, 5.979) (2.1277, 5.7018) (2.3611, 5.7018) knots 0 0 0 1 2 2 2
  spline S488 degree 2 poles (2.3611, 5.7018) (2.4437, 5.7018) (2.6042, 5.7391) (2.669, 5.7683) knots 0 0 0 1 2 2 2
  spline S489 degree 2 poles (2.669, 5.7683) (2.7371, 5.8007) (2.8311, 5.8574) (2.8619, 5.8833) knots 0 0 0 1 2 2 2
  line L399 (2.8619, 5.8833) -> (2.8765, 5.8833)
  line L400 (2.8765, 5.8833) -> (2.8765, 5.6078)
  spline S490 degree 2 poles (2.8765, 5.6078) (2.8327, 5.59) (2.6998, 5.5381) (2.6479, 5.5235) knots 0 0 0 1 2 2 2
  spline S491 degree 2 poles (2.6479, 5.5235) (2.575, 5.5025) (2.4551, 5.4814) (2.3643, 5.4814) knots 0 0 0 1 2 2 2
  spline S492 degree 2 poles (2.6577, 6.4328) (2.6544, 6.5349) (2.6123, 6.684) (2.5718, 6.7342) knots 0 0 0 1 2 2 2
  spline S493 degree 2 poles (2.5718, 6.7342) (2.528, 6.791) (2.3902, 6.8509) (2.2881, 6.8509) knots 0 0 0 1 2 2 2
  spline S494 degree 2 poles (2.2881, 6.8509) (2.1876, 6.8509) (2.0466, 6.791) (1.9883, 6.7326) knots 0 0 0 1 2 2 2
  spline S495 degree 2 poles (1.9883, 6.7326) (1.9316, 6.6727) (1.8732, 6.5284) (1.8651, 6.4328) knots 0 0 0 1 2 2 2
  line L401 (1.8651, 6.4328) -> (2.6577, 6.4328)
  spline S496 degree 2 poles (5.6155, 6.5138) (5.6155, 6.2399) (5.3935, 5.7991) (5.2071, 5.6759) knots 0 0 0 1 2 2 2
  spline S497 degree 2 poles (5.2071, 5.6759) (5.0547, 5.5803) (4.7419, 5.5154) (4.4988, 5.5154) knots 0 0 0 1 2 2 2
  line L402 (4.4988, 5.5154) -> (4.0385, 5.5154)
  line L403 (4.0385, 5.5154) -> (4.0385, 7.5154)
  line L404 (4.0385, 7.5154) -> (4.494, 7.5154)
  spline S498 degree 2 poles (4.494, 7.5154) (4.776, 7.5154) (5.0969, 7.4312) (5.2103, 7.3566) knots 0 0 0 1 2 2 2
  spline S499 degree 2 poles (5.2103, 7.3566) (5.4032, 7.2286) (5.6155, 6.8056) (5.6155, 6.5138) knots 0 0 0 1 2 2 2
  spline S500 degree 2 poles (5.3384, 6.5171) (5.3384, 6.7472) (5.186, 7.073) (5.0353, 7.1654) knots 0 0 0 1 2 2 2
  spline S501 degree 2 poles (5.0353, 7.1654) (4.9283, 7.2286) (4.6868, 7.2853) (4.5069, 7.2853) knots 0 0 0 1 2 2 2
  line L405 (4.5069, 7.2853) -> (4.3043, 7.2853)
  line L406 (4.3043, 7.2853) -> (4.3043, 5.7456)
  line L407 (4.3043, 5.7456) -> (4.5069, 5.7456)
  spline S502 degree 2 poles (4.5069, 5.7456) (4.6836, 5.7456) (4.951, 5.8023) (5.0596, 5.8785) knots 0 0 0 1 2 2 2
  spline S503 degree 2 poles (5.0596, 5.8785) (5.199, 5.9725) (5.3384, 6.2837) (5.3384, 6.5171) knots 0 0 0 1 2 2 2
  spline S504 degree 2 poles (6.6852, 5.4798) (6.4907, 5.4798) (6.1617, 5.6111) (6.0418, 5.7423) knots 0 0 0 1 2 2 2
  spline S505 degree 2 poles (6.0418, 5.7423) (5.9218, 5.872) (5.7906, 6.261) (5.7906, 6.5138) knots 0 0 0 1 2 2 2
  spline S506 degree 2 poles (5.7906, 6.5138) (5.7906, 6.765) (5.9186, 7.1378) (6.0401, 7.2756) knots 0 0 0 1 2 2 2
  spline S507 degree 2 poles (6.0401, 7.2756) (6.1601, 7.4101) (6.4875, 7.5511) (6.6901, 7.5511) knots 0 0 0 1 2 2 2
  spline S508 degree 2 poles (6.6901, 7.5511) (6.7906, 7.5511) (6.9672, 7.5219) (7.0418, 7.4992) knots 0 0 0 1 2 2 2
  spline S509 degree 2 poles (7.0418, 7.4992) (7.1066, 7.4782) (7.2411, 7.4182) (7.3076, 7.3825) knots 0 0 0 1 2 2 2
  line L408 (7.3076, 7.3825) -> (7.3076, 7.0616)
  line L409 (7.3076, 7.0616) -> (7.2865, 7.0616)
  spline S510 degree 2 poles (7.2865, 7.0616) (7.2508, 7.094) (7.1406, 7.1848) (7.0612, 7.2286) knots 0 0 0 1 2 2 2
  spline S511 degree 2 poles (7.0612, 7.2286) (6.985, 7.2707) (6.8051, 7.3242) (6.6884, 7.3242) knots 0 0 0 1 2 2 2
  spline S512 degree 2 poles (6.6884, 7.3242) (6.5604, 7.3242) (6.3319, 7.2188) (6.246, 7.1184) knots 0 0 0 1 2 2 2
  spline S513 degree 2 poles (6.246, 7.1184) (6.1617, 7.0162) (6.0677, 6.7067) (6.0677, 6.5138) knots 0 0 0 1 2 2 2
  spline S514 degree 2 poles (6.0677, 6.5138) (6.0677, 6.308) (6.1666, 6.0114) (6.2525, 5.9093) knots 0 0 0 1 2 2 2
  spline S515 degree 2 poles (6.2525, 5.9093) (6.3367, 5.8104) (6.562, 5.7099) (6.6884, 5.7099) knots 0 0 0 1 2 2 2
  spline S516 degree 2 poles (6.6884, 5.7099) (6.8035, 5.7099) (6.9996, 5.7667) (7.0758, 5.8088) knots 0 0 0 1 2 2 2
  spline S517 degree 2 poles (7.0758, 5.8088) (7.1487, 5.8509) (7.2573, 5.9385) (7.2881, 5.9692) knots 0 0 0 1 2 2 2
  line L410 (7.2881, 5.9692) -> (7.3076, 5.9692)
  line L411 (7.3076, 5.9692) -> (7.3076, 5.6516)
  spline S518 degree 2 poles (7.3076, 5.6516) (7.2411, 5.6208) (7.1244, 5.5641) (7.0418, 5.5381) knots 0 0 0 1 2 2 2
  spline S519 degree 2 poles (7.0418, 5.5381) (6.9542, 5.509) (6.8051, 5.4798) (6.6852, 5.4798) knots 0 0 0 1 2 2 2
  line L412 (-29.4137, 2.2225) -> (-28.7394, 4.2225)
  line L413 (-28.7394, 4.2225) -> (-28.412, 4.2225)
  line L414 (-28.412, 4.2225) -> (-27.7378, 2.2225)
  line L415 (-27.7378, 2.2225) -> (-28.0182, 2.2225)
  line L416 (-28.0182, 2.2225) -> (-28.1997, 2.7816)
  line L417 (-28.1997, 2.7816) -> (-28.9631, 2.7816)
  line L418 (-28.9631, 2.7816) -> (-29.1446, 2.2225)
  line L419 (-29.1446, 2.2225) -> (-29.4137, 2.2225)
  line L420 (-28.2727, 3.0086) -> (-28.5822, 3.9502)
  line L421 (-28.5822, 3.9502) -> (-28.8902, 3.0086)
  line L422 (-28.8902, 3.0086) -> (-28.2727, 3.0086)
  spline S520 degree 2 poles (-26.1122, 2.1885) (-26.2678, 2.1885) (-26.5255, 2.2841) (-26.6179, 2.3813) knots 0 0 0 1 2 2 2
  spline S521 degree 2 poles (-26.6179, 2.3813) (-26.7103, 2.4769) (-26.8124, 2.7719) (-26.8124, 2.9697) knots 0 0 0 1 2 2 2
  spline S522 degree 2 poles (-26.8124, 2.9697) (-26.8124, 3.1674) (-26.707, 3.4559) (-26.6179, 3.5531) knots 0 0 0 1 2 2 2
  spline S523 degree 2 poles (-26.6179, 3.5531) (-26.5287, 3.652) (-26.2646, 3.7573) (-26.1122, 3.7573) knots 0 0 0 1 2 2 2
  spline S524 degree 2 poles (-26.1122, 3.7573) (-25.989, 3.7573) (-25.7589, 3.6876) (-25.6697, 3.6423) knots 0 0 0 1 2 2 2
  line L423 (-25.6697, 3.6423) -> (-25.6697, 3.3586)
  line L424 (-25.6697, 3.3586) -> (-25.6843, 3.3586)
  spline S525 degree 2 poles (-25.6843, 3.3586) (-25.7119, 3.3813) (-25.7962, 3.4397) (-25.8561, 3.4705) knots 0 0 0 1 2 2 2
  spline S526 degree 2 poles (-25.8561, 3.4705) (-25.9096, 3.4964) (-26.0522, 3.5369) (-26.1171, 3.5369) knots 0 0 0 1 2 2 2
  spline S527 degree 2 poles (-26.1171, 3.5369) (-26.3132, 3.5369) (-26.5514, 3.2403) (-26.5514, 2.9697) knots 0 0 0 1 2 2 2
  spline S528 degree 2 poles (-26.5514, 2.9697) (-26.5514, 2.7055) (-26.3213, 2.4089) (-26.1171, 2.4089) knots 0 0 0 1 2 2 2
  spline S529 degree 2 poles (-26.1171, 2.4089) (-25.9939, 2.4089) (-25.7702, 2.511) (-25.6843, 2.5904) knots 0 0 0 1 2 2 2
  line L425 (-25.6843, 2.5904) -> (-25.6697, 2.5904)
  line L426 (-25.6697, 2.5904) -> (-25.6697, 2.3068)
  spline S530 degree 2 poles (-25.6697, 2.3068) (-25.707, 2.2889) (-25.8205, 2.2387) (-25.8658, 2.2274) knots 0 0 0 1 2 2 2
  spline S531 degree 2 poles (-25.8658, 2.2274) (-25.9307, 2.2079) (-26.0328, 2.1885) (-26.1122, 2.1885) knots 0 0 0 1 2 2 2
  line L427 (-24.2727, 2.2225) -> (-24.5255, 2.2225)
  line L428 (-24.5255, 2.2225) -> (-24.5255, 2.3878)
  spline S532 degree 2 poles (-24.5255, 2.3878) (-24.6422, 2.2857) (-24.8513, 2.1804) (-24.9809, 2.1804) knots 0 0 0 1 2 2 2
  spline S533 degree 2 poles (-24.9809, 2.1804) (-25.0782, 2.1804) (-25.2516, 2.2452) (-25.3148, 2.3149) knots 0 0 0 1 2 2 2
  spline S534 degree 2 poles (-25.3148, 2.3149) (-25.3796, 2.3846) (-25.4509, 2.5969) (-25.4509, 2.7492) knots 0 0 0 1 2 2 2
  line L429 (-25.4509, 2.7492) -> (-25.4509, 3.7233)
  line L430 (-25.4509, 3.7233) -> (-25.1981, 3.7233)
  line L431 (-25.1981, 3.7233) -> (-25.1981, 2.8675)
  spline S535 degree 2 poles (-25.1981, 2.8675) (-25.1981, 2.7476) (-25.1803, 2.5904) (-25.1495, 2.5321) knots 0 0 0 1 2 2 2
  spline S536 degree 2 poles (-25.1495, 2.5321) (-25.1187, 2.4737) (-25.0133, 2.4202) (-24.9145, 2.4202) knots 0 0 0 1 2 2 2
  spline S537 degree 2 poles (-24.9145, 2.4202) (-24.8221, 2.4202) (-24.613, 2.5256) (-24.5255, 2.6017) knots 0 0 0 1 2 2 2
  line L432 (-24.5255, 2.6017) -> (-24.5255, 3.7233)
  line L433 (-24.5255, 3.7233) -> (-24.2727, 3.7233)
  line L434 (-24.2727, 3.7233) -> (-24.2727, 2.2225)
  line L435 (-23.1106, 3.4526) -> (-23.1235, 3.4526)
  spline S538 degree 2 poles (-23.1235, 3.4526) (-23.1527, 3.4607) (-23.2159, 3.464) (-23.2597, 3.464) knots 0 0 0 1 2 2 2
  spline S539 degree 2 poles (-23.2597, 3.464) (-23.3618, 3.464) (-23.5628, 3.3748) (-23.6535, 3.2873) knots 0 0 0 1 2 2 2
  line L436 (-23.6535, 3.2873) -> (-23.6535, 2.2225)
  line L437 (-23.6535, 2.2225) -> (-23.9064, 2.2225)
  line L438 (-23.9064, 2.2225) -> (-23.9064, 3.7233)
  line L439 (-23.9064, 3.7233) -> (-23.6535, 3.7233)
  line L440 (-23.6535, 3.7233) -> (-23.6535, 3.4996)
  spline S540 degree 2 poles (-23.6535, 3.4996) (-23.5158, 3.6228) (-23.3099, 3.7233) (-23.2127, 3.7233) knots 0 0 0 1 2 2 2
  spline S541 degree 2 poles (-23.2127, 3.7233) (-23.1738, 3.7233) (-23.1349, 3.7201) (-23.1106, 3.7152) knots 0 0 0 1 2 2 2
  line L441 (-23.1106, 3.7152) -> (-23.1106, 3.4526)
  spline S542 degree 2 poles (-22.0782, 2.3813) (-22.109, 2.3586) (-22.2127, 2.2776) (-22.2613, 2.2533) knots 0 0 0 1 2 2 2
  spline S543 degree 2 poles (-22.2613, 2.2533) (-22.3278, 2.2176) (-22.4526, 2.1804) (-22.566, 2.1804) knots 0 0 0 1 2 2 2
  spline S544 degree 2 poles (-22.566, 2.1804) (-22.6584, 2.1804) (-22.8253, 2.25) (-22.8885, 2.3133) knots 0 0 0 1 2 2 2
  spline S545 degree 2 poles (-22.8885, 2.3133) (-22.9485, 2.3748) (-23.0214, 2.5564) (-23.0214, 2.6569) knots 0 0 0 1 2 2 2
  spline S546 degree 2 poles (-23.0214, 2.6569) (-23.0214, 2.8124) (-22.8902, 3.0329) (-22.7475, 3.0961) knots 0 0 0 1 2 2 2
  spline S547 degree 2 poles (-22.7475, 3.0961) (-22.6211, 3.1544) (-22.2775, 3.1982) (-22.0782, 3.2095) knots 0 0 0 1 2 2 2
  line L442 (-22.0782, 3.2095) -> (-22.0782, 3.2581)
  spline S548 degree 2 poles (-22.0782, 3.2581) (-22.0782, 3.3457) (-22.1317, 3.4543) (-22.1803, 3.4851) knots 0 0 0 1 2 2 2
  spline S549 degree 2 poles (-22.1803, 3.4851) (-22.2289, 3.5158) (-22.3683, 3.5353) (-22.4428, 3.5353) knots 0 0 0 1 2 2 2
  spline S550 degree 2 poles (-22.4428, 3.5353) (-22.5304, 3.5353) (-22.767, 3.4834) (-22.8853, 3.4332) knots 0 0 0 1 2 2 2
  line L443 (-22.8853, 3.4332) -> (-22.8999, 3.4332)
  line L444 (-22.8999, 3.4332) -> (-22.8999, 3.6909)
  spline S551 degree 2 poles (-22.8999, 3.6909) (-22.8302, 3.7103) (-22.5693, 3.759) (-22.4412, 3.759) knots 0 0 0 1 2 2 2
  spline S552 degree 2 poles (-22.4412, 3.759) (-22.2856, 3.759) (-22.0733, 3.7103) (-21.989, 3.6471) knots 0 0 0 1 2 2 2
  spline S553 degree 2 poles (-21.989, 3.6471) (-21.9064, 3.5855) (-21.8253, 3.3894) (-21.8253, 3.2484) knots 0 0 0 1 2 2 2
  line L445 (-21.8253, 3.2484) -> (-21.8253, 2.2225)
  line L446 (-21.8253, 2.2225) -> (-22.0782, 2.2225)
  line L447 (-22.0782, 2.2225) -> (-22.0782, 2.3813)
  line L448 (-22.0782, 2.592) -> (-22.0782, 3.0086)
  spline S554 degree 2 poles (-22.0782, 3.0086) (-22.1689, 3.0004) (-22.4428, 2.9729) (-22.5287, 2.947) knots 0 0 0 1 2 2 2
  spline S555 degree 2 poles (-22.5287, 2.947) (-22.6292, 2.9162) (-22.7605, 2.7881) (-22.7605, 2.6747) knots 0 0 0 1 2 2 2
  spline S556 degree 2 poles (-22.7605, 2.6747) (-22.7605, 2.545) (-22.6146, 2.4137) (-22.4752, 2.4137) knots 0 0 0 1 2 2 2
  spline S557 degree 2 poles (-22.4752, 2.4137) (-22.3569, 2.4137) (-22.1624, 2.5158) (-22.0782, 2.592) knots 0 0 0 1 2 2 2
  line L449 (-19.4574, 2.2225) -> (-19.7103, 2.2225)
  line L450 (-19.7103, 2.2225) -> (-19.7103, 2.3748)
  spline S558 degree 2 poles (-19.7103, 2.3748) (-19.7686, 2.3262) (-19.8545, 2.2614) (-19.9128, 2.2338) knots 0 0 0 1 2 2 2
  spline S559 degree 2 poles (-19.9128, 2.2338) (-19.9663, 2.2079) (-20.0814, 2.1804) (-20.1576, 2.1804) knots 0 0 0 1 2 2 2
  spline S560 degree 2 poles (-20.1576, 2.1804) (-20.2808, 2.1804) (-20.4882, 2.2825) (-20.5611, 2.3813) knots 0 0 0 1 2 2 2
  spline S561 degree 2 poles (-20.5611, 2.3813) (-20.6341, 2.4802) (-20.7151, 2.7719) (-20.7151, 2.9616) knots 0 0 0 1 2 2 2
  spline S562 degree 2 poles (-20.7151, 2.9616) (-20.7151, 3.1593) (-20.613, 3.4478) (-20.5239, 3.5564) knots 0 0 0 1 2 2 2
  spline S563 degree 2 poles (-20.5239, 3.5564) (-20.4412, 3.6536) (-20.2094, 3.7654) (-20.0814, 3.7654) knots 0 0 0 1 2 2 2
  spline S564 degree 2 poles (-20.0814, 3.7654) (-19.9696, 3.7654) (-19.8026, 3.7152) (-19.7103, 3.6633) knots 0 0 0 1 2 2 2
  line L451 (-19.7103, 3.6633) -> (-19.7103, 4.3116)
  line L452 (-19.7103, 4.3116) -> (-19.4574, 4.3116)
  line L453 (-19.4574, 4.3116) -> (-19.4574, 2.2225)
  line L454 (-19.7103, 2.5872) -> (-19.7103, 3.4543)
  spline S565 degree 2 poles (-19.7103, 3.4543) (-19.8043, 3.4996) (-19.9534, 3.5337) (-20.0393, 3.5337) knots 0 0 0 1 2 2 2
  spline S566 degree 2 poles (-20.0393, 3.5337) (-20.2338, 3.5337) (-20.4542, 3.2419) (-20.4542, 2.9664) knots 0 0 0 1 2 2 2
  spline S567 degree 2 poles (-20.4542, 2.9664) (-20.4542, 2.7006) (-20.2856, 2.4202) (-20.0992, 2.4202) knots 0 0 0 1 2 2 2
  spline S568 degree 2 poles (-20.0992, 2.4202) (-20.0004, 2.4202) (-19.7994, 2.511) (-19.7103, 2.5872) knots 0 0 0 1 2 2 2
  line L455 (-18.8334, 2.2225) -> (-19.0863, 2.2225)
  line L456 (-19.0863, 2.2225) -> (-19.0863, 3.7233)
  line L457 (-19.0863, 3.7233) -> (-18.8334, 3.7233)
  line L458 (-18.8334, 3.7233) -> (-18.8334, 2.2225)
  line L459 (-18.8156, 3.9729) -> (-19.1025, 3.9729)
  line L460 (-19.1025, 3.9729) -> (-19.1025, 4.2355)
  line L461 (-19.1025, 4.2355) -> (-18.8156, 4.2355)
  line L462 (-18.8156, 4.2355) -> (-18.8156, 3.9729)
  line L463 (-17.9987, 2.2225) -> (-18.3197, 2.2225)
  line L464 (-18.3197, 2.2225) -> (-18.3197, 2.605)
  line L465 (-18.3197, 2.605) -> (-17.9987, 2.605)
  line L466 (-17.9987, 2.605) -> (-17.9987, 2.2225)
  line L467 (-17.9987, 3.3408) -> (-18.3197, 3.3408)
  line L468 (-18.3197, 3.3408) -> (-18.3197, 3.7233)
  line L469 (-18.3197, 3.7233) -> (-17.9987, 3.7233)
  line L470 (-17.9987, 3.7233) -> (-17.9987, 3.3408)
  spline S569 degree 2 poles (-28.3034, -0.1823) (-28.3034, -0.3768) (-28.5822, -0.6539) (-28.7767, -0.6539) knots 0 0 0 1 2 2 2
  spline S570 degree 2 poles (-28.7767, -0.6539) (-28.9712, -0.6539) (-29.2483, -0.3768) (-29.2483, -0.1823) knots 0 0 0 1 2 2 2
  spline S571 degree 2 poles (-29.2483, -0.1823) (-29.2483, 0.0122) (-28.9712, 0.2893) (-28.7767, 0.2893) knots 0 0 0 1 2 2 2
  spline S572 degree 2 poles (-28.7767, 0.2893) (-28.5822, 0.2893) (-28.3034, 0.0122) (-28.3034, -0.1823) knots 0 0 0 1 2 2 2
  line L471 (-23.4137, -1.0705) -> (-22.7394, 0.9295)
  line L472 (-22.7394, 0.9295) -> (-22.412, 0.9295)
  line L473 (-22.412, 0.9295) -> (-21.7378, -1.0705)
  line L474 (-21.7378, -1.0705) -> (-22.0182, -1.0705)
  line L475 (-22.0182, -1.0705) -> (-22.1997, -0.5113)
  line L476 (-22.1997, -0.5113) -> (-22.9631, -0.5113)
  line L477 (-22.9631, -0.5113) -> (-23.1446, -1.0705)
  line L478 (-23.1446, -1.0705) -> (-23.4137, -1.0705)
  line L479 (-22.2727, -0.2844) -> (-22.5822, 0.6573)
  line L480 (-22.5822, 0.6573) -> (-22.8902, -0.2844)
  line L481 (-22.8902, -0.2844) -> (-22.2727, -0.2844)
  line L482 (-21.3099, -1.0705) -> (-21.5628, -1.0705)
  line L483 (-21.5628, -1.0705) -> (-21.5628, 1.0187)
  line L484 (-21.5628, 1.0187) -> (-21.3099, 1.0187)
  line L485 (-21.3099, 1.0187) -> (-21.3099, -1.0705)
  line L486 (-20.1495, 0.7756) -> (-20.1624, 0.7756)
  spline S573 degree 2 poles (-20.1624, 0.7756) (-20.1965, 0.7885) (-20.3229, 0.8112) (-20.3731, 0.8112) knots 0 0 0 1 2 2 2
  spline S574 degree 2 poles (-20.3731, 0.8112) (-20.532, 0.8112) (-20.6681, 0.6686) (-20.6681, 0.4806) knots 0 0 0 1 2 2 2
  line L487 (-20.6681, 0.4806) -> (-20.6681, 0.4304)
  line L488 (-20.6681, 0.4304) -> (-20.25, 0.4304)
  line L489 (-20.25, 0.4304) -> (-20.25, 0.2213)
  line L490 (-20.25, 0.2213) -> (-20.66, 0.2213)
  line L491 (-20.66, 0.2213) -> (-20.66, -1.0705)
  line L492 (-20.66, -1.0705) -> (-20.9128, -1.0705)
  line L493 (-20.9128, -1.0705) -> (-20.9128, 0.2213)
  line L494 (-20.9128, 0.2213) -> (-21.083, 0.2213)
  line L495 (-21.083, 0.2213) -> (-21.083, 0.4304)
  line L496 (-21.083, 0.4304) -> (-20.9128, 0.4304)
  line L497 (-20.9128, 0.4304) -> (-20.9128, 0.4806)
  spline S575 degree 2 poles (-20.9128, 0.4806) (-20.9128, 0.7496) (-20.6519, 1.0317) (-20.4088, 1.0317) knots 0 0 0 1 2 2 2
  spline S576 degree 2 poles (-20.4088, 1.0317) (-20.3391, 1.0317) (-20.2046, 1.0171) (-20.1495, 1.0073) knots 0 0 0 1 2 2 2
  line L498 (-20.1495, 1.0073) -> (-20.1495, 0.7756)
  spline S577 degree 2 poles (-19.2273, -0.9116) (-19.2581, -0.9343) (-19.3618, -1.0154) (-19.4104, -1.0397) knots 0 0 0 1 2 2 2
  spline S578 degree 2 poles (-19.4104, -1.0397) (-19.4769, -1.0753) (-19.6017, -1.1126) (-19.7151, -1.1126) knots 0 0 0 1 2 2 2
  spline S579 degree 2 poles (-19.7151, -1.1126) (-19.8075, -1.1126) (-19.9744, -1.0429) (-20.0376, -0.9797) knots 0 0 0 1 2 2 2
  spline S580 degree 2 poles (-20.0376, -0.9797) (-20.0976, -0.9181) (-20.1705, -0.7366) (-20.1705, -0.6361) knots 0 0 0 1 2 2 2
  spline S581 degree 2 poles (-20.1705, -0.6361) (-20.1705, -0.4805) (-20.0393, -0.2601) (-19.8966, -0.1969) knots 0 0 0 1 2 2 2
  spline S582 degree 2 poles (-19.8966, -0.1969) (-19.7702, -0.1385) (-19.4266, -0.0948) (-19.2273, -0.0834) knots 0 0 0 1 2 2 2
  line L499 (-19.2273, -0.0834) -> (-19.2273, -0.0348)
  spline S583 degree 2 poles (-19.2273, -0.0348) (-19.2273, 0.0527) (-19.2808, 0.1613) (-19.3294, 0.1921) knots 0 0 0 1 2 2 2
  spline S584 degree 2 poles (-19.3294, 0.1921) (-19.378, 0.2229) (-19.5174, 0.2423) (-19.5919, 0.2423) knots 0 0 0 1 2 2 2
  spline S585 degree 2 poles (-19.5919, 0.2423) (-19.6795, 0.2423) (-19.9161, 0.1905) (-20.0344, 0.1402) knots 0 0 0 1 2 2 2
  line L500 (-20.0344, 0.1402) -> (-20.049, 0.1402)
  line L501 (-20.049, 0.1402) -> (-20.049, 0.3979)
  spline S586 degree 2 poles (-20.049, 0.3979) (-19.9793, 0.4174) (-19.7184, 0.466) (-19.5903, 0.466) knots 0 0 0 1 2 2 2
  spline S587 degree 2 poles (-19.5903, 0.466) (-19.4347, 0.466) (-19.2224, 0.4174) (-19.1381, 0.3542) knots 0 0 0 1 2 2 2
  spline S588 degree 2 poles (-19.1381, 0.3542) (-19.0555, 0.2926) (-18.9744, 0.0965) (-18.9744, -0.0445) knots 0 0 0 1 2 2 2
  line L502 (-18.9744, -0.0445) -> (-18.9744, -1.0705)
  line L503 (-18.9744, -1.0705) -> (-19.2273, -1.0705)
  line L504 (-19.2273, -1.0705) -> (-19.2273, -0.9116)
  line L505 (-19.2273, -0.7009) -> (-19.2273, -0.2844)
  spline S589 degree 2 poles (-19.2273, -0.2844) (-19.318, -0.2925) (-19.5919, -0.3201) (-19.6778, -0.346) knots 0 0 0 1 2 2 2
  spline S590 degree 2 poles (-19.6778, -0.346) (-19.7783, -0.3768) (-19.9096, -0.5048) (-19.9096, -0.6183) knots 0 0 0 1 2 2 2
  spline S591 degree 2 poles (-19.9096, -0.6183) (-19.9096, -0.7479) (-19.7637, -0.8792) (-19.6244, -0.8792) knots 0 0 0 1 2 2 2